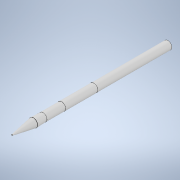
# Autodesk Inventor part: hude
Saved by Autodesk Inventor 2020.2 (Build 242310000, 310)
## iProperties
Created: 2020-10-31
Part Number: hude
Material: 一般
Document SubType Name: Modeling
Designer: touhu_zn72wdq
Density: 1 g/cm^3
Appearance: 既定
Author: touhu_zn72wdq
Autodesk Inventor part; units mm, degrees
ref_plane "YZ Plane" through (0, 0, 0) normal (1, 0, 0) x (0, 1, 0)
ref_plane "XZ Plane" through (0, 0, 0) normal (0, 1, 0) x (-1, 0, 0)
ref_plane "XY Plane" through (0, 0, 0) normal (0, 0, 1) x (1, 0, 0)
sketch "スケッチ5" plane through (0, 0, 0) normal (0, 0, 1) x (1, 0, 0)
  circle A0 centre (0, 0) radius 6.25
  dimension "d14" = 12.5
  constraints: 1 centre point, 1 coincident
  measures "d14" diameter of A0
extrude "押し出し5" add sketch "スケッチ5" along normal blind 115
sketch "スケッチ6" plane through (0, 0, 115) normal (0, 0, 1) x (1, 0, 0)
  circle A0 centre (0, 0) radius 6.35
  dimension "d17" = 12.7
  constraints: 1 centre point, 1 coincident
  measures "d17" diameter of A0
extrude "押し出し6" add sketch "スケッチ6" along normal blind 50
sketch "スケッチ7" plane through (0, 0, 165) normal (0, 0, 1) x (1, 0, 0)
  circle A0 centre (0, 0) radius 6.25
  dimension "d20" = 12.5
  constraints: 1 centre point, 1 coincident
  measures "d20" diameter of A0
extrude "押し出し7" add sketch "スケッチ7" along normal blind 29
sketch "スケッチ8" plane through (0, 0, 194) normal (0, 0, 1) x (1, 0, 0)
  circle A0 centre (0, 0) radius 6.2
  dimension "d23" = 12.4
  constraints: 1 centre point, 1 coincident
  measures "d23" diameter of A0
extrude "押し出し8" add sketch "スケッチ8" along normal blind 15 draft 2
sketch "スケッチ9" plane through (0, 0, 209) normal (0, 0, 1) x (1, 0, 0)
  circle A0 centre (0, 0) radius 6.7238
  constraints: 1 centre point, 1 coincident
extrude "押し出し9" add sketch "スケッチ9" along normal blind 33 draft -10
fillet "フィレット3" radius 2 1 edges at (-6.7238, 0, 209)
